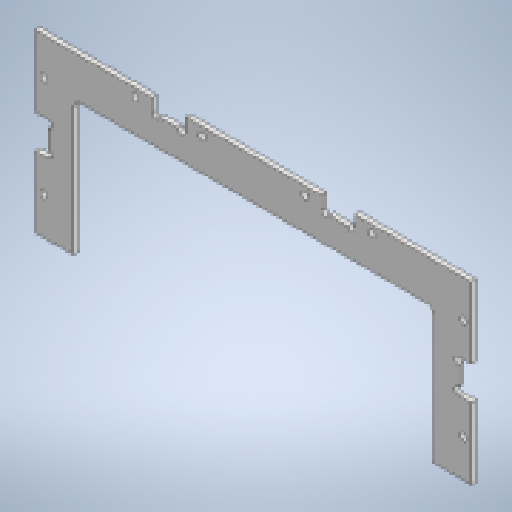
# Autodesk Inventor part: huta
Saved by Autodesk Inventor 2024 (Build 280153000, 153)
## iProperties
Created: 2024-06-06
Part Number: huta
Material: 一般
Document SubType Name: Modeling
Designer: right
Density: 1 g/cm^3
Appearance: 既定
Author: right
Autodesk Inventor part; units mm, degrees
ref_plane "YZ Plane" through (0, 0, 0) normal (1, 0, 0) x (0, 1, 0)
ref_plane "XZ Plane" through (0, 0, 0) normal (0, 1, 0) x (-1, 0, 0)
ref_plane "XY Plane" through (0, 0, 0) normal (0, 0, 1) x (1, 0, 0)
sketch "スケッチ1" plane through (0, 0, 0) normal (0, 0, 1) x (1, 0, 0)
  line L0 (64.854, -28.5883) -> (60.854, -28.5883) projected
  arc A0 (60.854, -26.3883) -> (60.854, -28.5883) centre (60.854, -27.4883) ccw projected
  line L1 (60.854, -26.3883) -> (60.854, -20.7883) projected
  arc A1 (60.854, -18.5883) -> (60.854, -20.7883) centre (60.854, -19.6883) ccw projected
  line L2 (60.854, -18.5883) -> (64.854, -18.5883) projected
  line L3 (64.854, -18.5883) -> (64.854, 2.5169) projected
  line L4 (30.25, 2.5169) -> (64.854, 2.5169) projected
  line L5 (30.25, 2.5169) -> (30.25, -1.5) projected
  arc A2 (28.05, -1.5) -> (30.25, -1.5) centre (29.15, -1.5) ccw projected
  line L6 (28.05, -1.5) -> (22.45, -1.5) projected
  arc A3 (20.25, -1.5) -> (22.45, -1.5) centre (21.35, -1.5) ccw projected
  line L7 (20.25, -1.5) -> (20.25, 2.5169) projected
  line L8 (-20.25, 2.5169) -> (20.25, 2.5169) projected
  line L9 (-20.25, 2.5169) -> (-20.25, -1.5) projected
  arc A4 (-22.45, -1.5) -> (-20.25, -1.5) centre (-21.35, -1.5) ccw projected
  line L10 (-22.45, -1.5) -> (-28.05, -1.5) projected
  arc A5 (-30.25, -1.5) -> (-28.05, -1.5) centre (-29.15, -1.5) ccw projected
  line L11 (-30.25, -1.5) -> (-30.25, 2.5169) projected
  line L12 (-30.25, 2.5169) -> (-64.854, 2.5169) projected
  line L13 (-64.854, 2.5169) -> (-64.854, -18.5883) projected
  line L14 (-64.854, -18.5883) -> (-60.854, -18.5883) projected
  arc A6 (-60.854, -20.7883) -> (-60.854, -18.5883) centre (-60.854, -19.6883) ccw projected
  line L15 (-60.854, -20.7883) -> (-60.854, -26.3883) projected
  arc A7 (-60.854, -28.5883) -> (-60.854, -26.3883) centre (-60.854, -27.4883) ccw projected
  line L16 (-60.854, -28.5883) -> (-64.854, -28.5883) projected
  line L17 (-64.854, -28.5883) -> (-64.854, -49.6935) projected
  line L18 (-64.854, -49.6935) -> (64.854, -49.6935) projected
  line L19 (64.854, -49.6935) -> (64.854, -28.5883) projected
  circle A8 centre (-15.25, 0) radius 1.1 projected
  circle A9 centre (15.25, 0) radius 1.1 projected
  circle A10 centre (35.25, 0) radius 1.1 projected
  circle A11 centre (-35.25, 0) radius 1.1 projected
  circle A12 centre (-45.5, -44.6935) radius 1.6 projected
  circle A13 centre (0, -44.6935) radius 1.6 projected
  circle A14 centre (45.5, -44.6935) radius 1.6 projected
  arc A15 (-50.5, -17.4831) -> (-50.5, -23.4831) centre (-50.5, -20.4831) ccw projected
  line L20 (50.5, -17.4831) -> (-50.5, -17.4831) projected
  arc A16 (50.5, -23.4831) -> (50.5, -17.4831) centre (50.5, -20.4831) ccw projected
  line L21 (-50.5, -23.4831) -> (50.5, -23.4831) projected
  circle A17 centre (62.354, -8.5883) radius 1.1 projected
  circle A18 centre (-62.354, -8.5883) radius 1.1 projected
  circle A19 centre (-62.354, -38.5883) radius 1.1 projected
  circle A20 centre (62.354, -38.5883) radius 1.1 projected
  line L22 (-15.8223, -11.5529) -> (3.1777, -11.5529) projected
  line L23 (53.5, -9.5529) -> (-53.5, -9.5529)
  line L24 (53.5, -9.5529) -> (53.5, -49.6935)
  line L25 (-53.5, -9.5529) -> (-53.5, -49.6935)
  point P0 (0, 0)
  dimension "d0" = 2
  constraints: 6 end point, 2 point on line, 2 tangent, 2 vertical, 1 horizontal
  measures "d0" distance between parallel lines of L23 L22
extrude "押し出し1" add sketch "スケッチ1" along normal blind 1.5 contours L19 L18 L24 L23 L25 L17 L16 A7 L15 A6 L14 L13 L12 L11 A5 L10 A4 L9 L8 L7 A3 L6 A2 L5 L4 L3 L2 A1 L1 A0 L0
fillet "フィレット1" radius 2 2 edges at (-53.5, -9.5529, 0.75) (53.5, -9.5529, 0.75)
